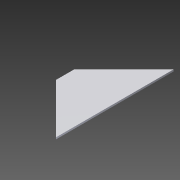
# Autodesk Inventor part: top short
Saved by Autodesk Inventor 2015 (Build 190159000, 159)
## iProperties
Created: 2019-04-10
Part Number: top short
Material: Generic
Document SubType Name: Modeling
Designer: Raptor
Density: 1 g/cm^3
Appearance: Snow
Author: Raptor
Autodesk Inventor part; units mm, degrees
ref_plane "YZ Plane" through (0, 0, 0) normal (1, 0, 0) x (0, 1, 0)
ref_plane "XZ Plane" through (0, 0, 0) normal (0, 1, 0) x (-1, 0, 0)
ref_plane "XY Plane" through (0, 0, 0) normal (0, 0, 1) x (1, 0, 0)
sketch "Sketch1" plane through (0, 0, 0) normal (0, 1, 0) x (-1, 0, 0)
  line L0 (0, 0) -> (0, -1300)
  line L1 (0, -1300) -> (550, -750)
  line L2 (550, -750) -> (550, -550)
  line L3 (0, 0) -> (550, -550)
  dimension "d0" = 45
  dimension "d1" = 45
  dimension "d3" = 1300
  dimension "d6" = 550
  constraints: 8 end point, 1 parallel, 1 vertical
  measures "d0" angle of L0 L3
  measures "d1" angle of L1 L0
  measures "d3" distance of L0.start L0.end
  measures "d6" distance between parallel lines of L0 L2
extrude "Extrusion1" add sketch "Sketch1" along normal blind 20
body "Solid1"
